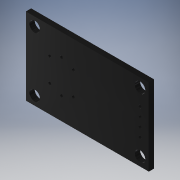
# Autodesk Inventor part: Platine
Saved by Autodesk Inventor 2019 (Build 230136000, 136)
## iProperties
Created: 2019-06-05
Part Number: Platine
Material: LCP-Kunststoff
Document SubType Name: Modeling
Designer: manue
Density: 1.626 g/cm^3
Appearance: Glatt - Schwarz
Author: manue
Autodesk Inventor part; units mm, degrees
ref_plane "YZ Plane" through (0, 0, 0) normal (1, 0, 0) x (0, 1, 0)
ref_plane "XZ Plane" through (0, 0, 0) normal (0, 1, 0) x (-1, 0, 0)
ref_plane "XY Plane" through (0, 0, 0) normal (0, 0, 1) x (1, 0, 0)
sketch "Skizze1" plane through (0, 0, 0) normal (0, 0, 1) x (1, 0, 0)
  line L0 (0, 0) -> (35, 0)
  line L1 (35, 0) -> (35, 22)
  line L2 (35, 22) -> (0, 22)
  line L3 (0, 22) -> (0, 0)
  dimension "d0" = 35
  dimension "d1" = 22
  constraints: 8 end point, 2 parallel, 1 horizontal, 1 perpendicular
  measures "d0" distance of L2.end L1.end
  measures "d1" distance of L1.end L0.end
extrude "Extrusion1" add sketch "Skizze1" along normal blind 1.5
sketch "Skizze2" plane through (0, 0, 1.5) normal (0, 0, 1) x (1, 0, 0)
  line L0 (0, 0) -> (35, 0) construction
  line L1 (35, 0) -> (35, 22) construction
  line L2 (35, 22) -> (0, 22) construction
  line L3 (0, 22) -> (0, 0) construction
  line L4 (35, 0) -> (35, 22) construction
  line L5 (35, 11) -> (0, 11) construction
  line L6 (0, 22) -> (0, 0) construction
  line L7 (0, 0) -> (35, 0) construction
  line L8 (17.5, 0) -> (17.5, 22) construction
  line L9 (35, 22) -> (0, 22) construction
  point P0 (32.5, 19.5)
  point P1 (32.5, 2.5)
  point P2 (2.5, 19.5)
  point P3 (2.5, 2.5)
  dimension "d4" = 2.5
  dimension "d5" = 2.5
  constraints: 4 end point, 4 midpoint, 3 symmetric about line
  measures "d4" distance from line of L1 point (32.5, 19.5)
  measures "d5" distance from line of L2 point (32.5, 19.5)
hole "Bohrung1" at (32.5, 19.5, 1.5) at (32.5, 2.5, 1.5) at (2.5, 2.5, 1.5) at (2.5, 19.5, 1.5) direction (0, 0, -1) diameter 3 end through all
sketch "Skizze3" plane through (0, 0, 1.5) normal (0, 0, 1) x (1, 0, 0)
  line L0 (35, 0) -> (35, 22) construction
  circle A0 centre (32.5, 2.5) radius 1.5 construction
  line L1 (32.5, 9.73) -> (32.5, 12.27) construction
  point P0 (0, 0)
  point P1 (32.5, 7.19)
  point P2 (32.5, 14.81)
  point P3 (32.5, 11)
  point P4 (35, 11)
  dimension "d15" = 2.54
  constraints: 2 end point, 2 midpoint, 2 vertical, 1 horizontal alignment, 1 vertical alignment, 3 other
  measures "d15" distance of point (32.5, 7.19) L1.start
hole "Bohrung2" at (32.5, 7.19, 1.5) at (32.5, 9.73, 1.5) at (32.5, 12.27, 1.5) at (32.5, 14.81, 1.5) direction (0, 0, -1) diameter 0.8 end through all
sketch "Skizze4" plane through (0, 0, 0) normal (0, 0, -1) x (-1, 0, 0)
  line L0 (0, 22) -> (0, 0) construction
  line L1 (0, 11) -> (-35, 11) construction
  line L2 (-35, 0) -> (-35, 22) construction
  line L3 (-10.1588, 15.75) -> (-10.1588, 6.25) construction
  point P0 (-6.8, 14.3588)
  point P1 (-13.5175, 14.3588)
  point P2 (-6.8, 7.6412)
  point P3 (-13.5175, 7.6412)
  dimension "d27" = 6.7175
  dimension "d29" = 6.7175
  dimension "d30" = 3.6355
  dimension "d31" = 6.8
  constraints: 4 end point, 4 symmetric about line, 2 midpoint, 1 horizontal alignment, 1 vertical
  measures "d27" distance of point (-13.518, 14.359) point (-6.8, 14.359)
  measures "d29" distance of point (-6.8, 7.641) point (-6.8, 14.359)
  measures "d30" distance of L3.start point (-6.8, 14.359)
  measures "d31" distance from line of L0 point (-6.8, 7.641)
hole "Bohrung3" at (6.8, 14.3588, 0) at (10.1588, 15.75, 0) at (13.5175, 14.3588, 0) at (6.8, 7.6412, 0) at (10.1588, 6.25, 0) at (13.5175, 7.6412, 0) direction (0, 0, 1) diameter 0.8 end through all
equation "\"d29\" = d27"
